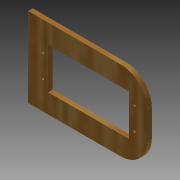
# Autodesk Inventor part: segment1c
Saved by Autodesk Inventor 2013 (Build 170138000, 138)
## iProperties
Created: 2014-10-10
Part Number: segment1c
Material: Plywood, Finish
Document SubType Name: Modeling
Designer: Masta
Density: 0.552 g/cm^3
Mass: 56.9255 g
Surface Area: 405.946 cm^2
Volume: 103.126 cm^3
Author: Masta
Autodesk Inventor part; units mm, degrees
ref_plane "YZ Plane" through (0, 0, 0) normal (1, 0, 0) x (0, 1, 0)
ref_plane "XZ Plane" through (0, 0, 0) normal (0, 1, 0) x (-1, 0, 0)
ref_plane "XY Plane" through (0, 0, 0) normal (0, 0, 1) x (1, 0, 0)
sketch "Sketch1" plane through (0, 0, 0) normal (0, 1, 0) x (-1, 0, 0)
  line L0 (0, 0) -> (-16.25, 0)
  line L1 (0, 0) -> (44.75, 0)
  line L2 (300, 0) -> (330, 0) construction
  line L3 (330, 30) -> (-30, 30) construction
  line L4 (-16.25, 15.5) -> (44.75, 15.5)
  line L5 (44.75, 15.5) -> (44.75, 0)
  line L6 (44.75, -15.5) -> (-16.25, -15.5)
  line L7 (-16.25, -15.5) -> (-16.25, 0)
  line L8 (-16.25, 15.5) -> (44.75, -15.5) construction
  line L9 (44.75, 15.5) -> (-16.25, -15.5) construction
  line L10 (-20.25, 8.5) -> (48.75, 8.5) construction
  line L11 (48.75, 8.5) -> (48.75, -8.5) construction
  line L12 (48.75, -8.5) -> (-20.25, -8.5) construction
  line L13 (-20.25, -8.5) -> (-20.25, 8.5) construction
  line L14 (-20.25, 8.5) -> (48.75, -8.5) construction
  line L15 (48.75, 8.5) -> (-20.25, -8.5) construction
  line L16 (-30, 0) -> (-30, 30)
  line L17 (330, 0) -> (330, 30) construction
  line L18 (44.75, 0) -> (300, 0) construction
  line L19 (44.75, 0) -> (44.75, -15.5)
  line L20 (-16.25, 0) -> (-30, 0)
  line L21 (-16.25, 0) -> (-16.25, 15.5)
  line L22 (300, 0) -> (300, 18.5) construction
  line L23 (0, 0) -> (-30, 0) construction
  line L24 (44.75, 0) -> (59.75, 0)
  line L25 (59.75, 0) -> (59.75, 30)
  line L26 (-30, 30) -> (59.75, 30)
  point P0 (14.25, 0)
  point P1 (14.25, 0)
  point P2 (285, 0)
  dimension "d0" = 300
  dimension "d5" = 61
  dimension "d6" = 31
  dimension "d7" = 69
  dimension "d8" = 17
  dimension "d9" = 16.25
  dimension "d10" = 30
  dimension "d11" = 30
  dimension "d20" = 18.5
  dimension "d21" = 15
  dimension "d29" = 15
  constraints: 54 end point, 10 parallel, 6 collinear, 6 perpendicular, 5 coincident, 5 midpoint, 5 point on line, 4 horizontal
  measures "d0" distance of L0.start L2.start
  measures "d5" distance of L6.start L6.end
  measures "d6" distance of L4.end L6.start
  measures "d7" distance of L11.end L12.end
  measures "d8" distance of L10.end L11.end
  measures "d9" distance from line of L7 point (0, 0)
  measures "d10" distance of L16.start L3.end
  measures "d11" distance of L2.end L3.start
  measures "d20" distance of L22.start L22.end
  measures "d21" distance of L22.start point (285, 0)
  measures "d29" distance of L1.end L24.end
extrude "Extrusion1" add sketch "Sketch1" along normal blind 3.5 contours L20 L16 L26 L25 L24 L5 L4 L21
hole "Hole1" at (20.25, 0, 8.5) at (-48.75, 0, 8.5) direction (0, 1, 0) diameter 2 end through all
fillet "Fillet1" radius 20 1 edges at (30, 1.75, 30)
mirror "Mirror1" about plane through (30, 0, 0) normal (0, 0, -1)
body "Solid1"
